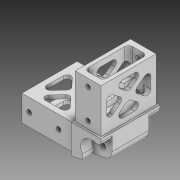
# Autodesk Inventor part: 254 Billet Bottom Block
Saved by Autodesk Inventor 2021 (Build 250183000, 183)
## iProperties
Created: 2021-03-21
Part Number: 254 Billet Bottom Block
Material: Generic
Document SubType Name: Modeling
Density: 1 g/cm^3
Appearance: Default
Autodesk Inventor part; units mm, degrees
ref_plane "YZ Plane" through (0, 0, 0) normal (1, 0, 0) x (0, 1, 0)
ref_plane "XZ Plane" through (0, 0, 0) normal (0, 1, 0) x (-1, 0, 0)
ref_plane "XY Plane" through (0, 0, 0) normal (0, 0, 1) x (1, 0, 0)
sketch "Sketch1" plane through (0, 0, 0) normal (0, 0, 1) x (1, 0, 0)
  line L0 (-71.4375, 14.2875) -> (-26.9875, 14.2875)
  line L1 (-26.9875, 14.2875) -> (-26.9875, -11.1125)
  line L2 (-26.9875, -11.1125) -> (-71.4375, -11.1125)
  line L3 (-71.4375, -11.1125) -> (-71.4375, 14.2875)
  line L4 (-26.9875, 14.2875) -> (-1.5875, 14.2875)
  line L5 (-1.5875, 14.2875) -> (-1.5875, 52.3875)
  line L6 (-1.5875, 52.3875) -> (-26.9875, 52.3875)
  line L7 (-26.9875, 52.3875) -> (-26.9875, 14.2875)
  circle A0 centre (-39.6875, 1.5875) radius 2.0193
  circle A1 centre (-65.0875, 1.5875) radius 2.0193
  circle A2 centre (-14.2875, 20.6375) radius 2.0193
  circle A3 centre (-14.2875, 46.0375) radius 2.0193
  line L8 (0, 0) -> (0, 64.1465) construction
  circle A4 centre (-9.525, 0) radius 9.525 construction
  line L9 (-31.5382, -9.525) -> (14.8852, -9.525) construction
  circle A5 centre (-9.525, 0) radius 2.5527
  arc A6 (-8.1574, -7.8188) -> (-1.5875, 0) centre (-9.525, 0) ccw
  line L10 (-1.5875, 14.2875) -> (-1.5875, 0)
  line L11 (-26.9875, -11.1125) -> (-8.1574, -7.8188)
  line L12 (-25.4, 52.3875) -> (-25.4, 17.5252)
  line L13 (-25.4, 17.5252) -> (-25.4, 14.2875)
  line L14 (-71.4375, 12.7) -> (-26.9875, 12.7)
  line L15 (-3.175, 14.2875) -> (-3.175, 52.3875)
  line L16 (-26.9875, -9.525) -> (-71.4375, -9.525)
  point P0 (-71.4375, 1.5875)
  point P1 (-14.2875, 14.2875)
  dimension "d0" = 4.0386
  dimension "d3" = 25.4
  dimension "d8" = 6.35
  dimension "d9" = 12.7
  dimension "d10" = 25.4
  dimension "d13" = 25.4
  dimension "d18" = 6.35
  dimension "d19" = 6.35
  dimension "d20" = 19.05
  dimension "d21" = 1.5875
  dimension "d22" = 1.5875
  dimension "d23" = 5.1054
  dimension "d24" = 15.875
  dimension "d25" = 1.5875
  dimension "d26" = 1.5875
  dimension "d27" = 1.5875
  dimension "d28" = 1.5875
  constraints: 34 end point, 9 point on line, 7 centre point, 6 perpendicular, 4 horizontal, 4 parallel, 4 tangent, 3 vertical, 2 horizontal alignment, 2 midpoint, 2 point on circle, 1 coincident, 1 equal radius, 1 vertical alignment, 4 other
  measures "d0" diameter of A0
  measures "d3" distance of A0.centre A1.centre
  measures "d8" distance from line of A1.centre L3
  measures "d9" distance from line of L1 A0.centre
  measures "d10" distance of L2.end L0.start
  measures "d13" distance of A2.centre A3.centre
  measures "d18" distance from line of L4 A2.centre
  measures "d19" distance from line of L6 A3.centre
  measures "d20" diameter of A4
  measures "d21" distance between parallel lines of L2 L9
  measures "d22" distance between parallel lines of L8 L5
  measures "d23" diameter of A5
  measures "d24" diameter of A6
  measures "d25" distance between parallel lines of L7 L12
  measures "d26" distance between parallel lines of L0 L14
  measures "d27" distance between parallel lines of L2 L16
  measures "d28" distance between parallel lines of L5 L15
extrude "Extrusion1" add sketch "Sketch1" along normal mid plane 50.8 contours L4 L10 A6 L11 L1 | L14 L1 L16 L3 | L13 L12 L6 L15 L4
sketch "Sketch2" plane through (0, 0, 25.4) normal (0, 0, 1) x (1, 0, 0)
  circle A0 centre (-9.525, 0) radius 2.5527 projected
  circle A1 centre (-9.525, 0) radius 9.6044
  point P0 (0, 0)
  dimension "d31" = 19.2087
  constraints: 1 centre point, 1 coincident
  measures "d31" diameter of A1
extrude "Extrusion2" cut sketch "Sketch2" against normal blind 9.525
mirror "Mirror1" about plane through (0, 0, 0) normal (0, 0, 1) of "Extrusion2"
fillet "Fillet1" radius 3.175 4 edges at (-13.4839, -8.7505, 20.6375) (-1.5875, 5.4074, 20.6375) (-1.5875, 5.4074, -20.6375) (-13.4839, -8.7505, -20.6375)
sketch "Sketch3" plane through (-71.4375, -9.525, 25.4) normal (-1, 0, 0) x (0, 0, 1)
  line L0 (-50.8, 0) -> (0, 0) projected
  line L1 (0, 22.225) -> (0, 0) projected
  line L2 (-50.8, 22.225) -> (0, 22.225) projected
  line L3 (-50.8, 0) -> (-50.8, 22.225) projected
  line L4 (-44.45, 19.05) -> (-6.35, 19.05)
  line L5 (-6.35, 19.05) -> (-6.35, 3.175)
  line L6 (-6.35, 3.175) -> (-44.45, 3.175)
  line L7 (-44.45, 3.175) -> (-44.45, 19.05)
  line L8 (-49.2125, 22.225) -> (-49.2125, 0)
  line L9 (0, 0) -> (-50.8, 0) projected
  line L10 (-50.8, 22.225) -> (0, 22.225) projected
  line L11 (-1.5875, 22.225) -> (-1.5875, 0)
  point P0 (-25.4, 9.525)
  point P1 (-49.2125, 0)
  dimension "d35" = 6.35
  dimension "d36" = 6.35
  dimension "d37" = 3.175
  dimension "d38" = 3.175
  dimension "d49" = 1.5875
  dimension "d50" = 1.5875
  constraints: 12 end point, 4 point on line, 3 parallel, 1 horizontal, 1 perpendicular, 1 vertical
  measures "d35" distance between parallel lines of L1 L5
  measures "d36" distance between parallel lines of L3 L7
  measures "d37" distance between parallel lines of L2 L4
  measures "d38" distance between parallel lines of L0 L6
  measures "d49" distance between parallel lines of L3 L8
  measures "d50" distance between parallel lines of L1 L11
extrude "Extrusion3" cut sketch "Sketch3" against normal up to surface (44.45 mm away) contours L3 L2 L8 L0 | L11 L2 L1 L0 | L4 L5 L6 L7
sketch "Sketch4" plane through (-25.4, 52.3875, 25.4) normal (0, 1, 0) x (1, 0, 0)
  line L0 (0, 50.8) -> (0, 0) projected
  line L1 (22.225, 0) -> (0, 0) projected
  line L2 (22.225, 50.8) -> (22.225, 0) projected
  line L3 (0, 50.8) -> (22.225, 50.8) projected
  line L4 (19.05, 6.35) -> (3.175, 6.35)
  line L5 (3.175, 6.35) -> (3.175, 44.45)
  line L6 (3.175, 44.45) -> (19.05, 44.45)
  line L7 (19.05, 44.45) -> (19.05, 6.35)
  line L8 (22.225, 49.2125) -> (0, 49.2125)
  line L9 (22.225, 1.5875) -> (0, 1.5875)
  point P0 (25.4, 25.4)
  dimension "d41" = 3.175
  dimension "d42" = 3.175
  dimension "d43" = 6.35
  dimension "d44" = 6.35
  dimension "d45" = 1.5875
  dimension "d46" = 1.5875
  constraints: 12 end point, 4 point on line, 3 perpendicular, 2 parallel, 1 horizontal
  measures "d41" distance between parallel lines of L2 L7
  measures "d42" distance between parallel lines of L0 L5
  measures "d43" distance between parallel lines of L1 L4
  measures "d44" distance between parallel lines of L3 L6
  measures "d45" distance between parallel lines of L1 L9
  measures "d46" distance between parallel lines of L3 L8
extrude "Extrusion4" cut sketch "Sketch4" against normal up to surface (38.1 mm away) contours L3 L2 L8 L0 | L9 L2 L1 L0 | L4 L5 L6 L7
sketch "Sketch5" plane through (-71.4375, 12.7, 23.8125) normal (0, 1, 0) x (1, 0, 0)
  line L0 (0, 0) -> (44.45, 0) projected
  line L1 (44.45, 47.625) -> (44.45, 0) projected
  line L2 (44.45, 47.625) -> (0, 47.625) projected
  line L3 (0, 47.625) -> (0, 0) projected
  line L4 (44.45, 4.7625) -> (44.45, 42.8625) projected
  line L5 (0, 42.8625) -> (44.45, 42.8625) projected
  line L6 (0, 4.7625) -> (0, 42.8625) projected
  line L7 (0, 4.7625) -> (44.45, 4.7625) projected
  line L8 (4.7625, 0) -> (4.7625, 47.625)
  line L9 (39.6875, 0) -> (39.6875, 47.625)
  line L10 (44.45, 47.625) -> (0, 47.625) projected
  line L11 (0, 4.7625) -> (44.45, 4.7625) projected
  line L12 (39.6875, 4.7625) -> (4.7625, 42.8625) construction
  line L13 (41.4428, 6.3716) -> (6.5178, 44.4716)
  line L14 (3.0072, 41.2534) -> (37.9322, 3.1534)
  arc A0 (37.9322, 3.1534) -> (41.4428, 6.3716) centre (39.6875, 4.7625) ccw
  arc A1 (6.5178, 44.4716) -> (3.0072, 41.2534) centre (4.7625, 42.8625) ccw
  line L15 (4.7625, 4.7625) -> (39.6875, 42.8625) construction
  line L16 (6.5178, 3.1534) -> (41.4428, 41.2534)
  line L17 (37.9322, 44.4716) -> (3.0072, 6.3716)
  arc A2 (3.0072, 6.3716) -> (6.5178, 3.1534) centre (4.7625, 4.7625) ccw
  arc A3 (41.4428, 41.2534) -> (37.9322, 44.4716) centre (39.6875, 42.8625) ccw
  point P0 (71.4375, 23.8125)
  point P1 (22.225, 23.8125)
  point P2 (22.225, 23.8125)
  point P3 (22.225, 27.3365)
  point P4 (36.4572, 42.8625)
  point P5 (7.9928, 42.8625)
  point P6 (39.6875, 39.3385)
  point P7 (25.4553, 23.8125)
  point P8 (39.6875, 8.2865)
  point P9 (22.225, 20.2885)
  point P10 (7.9928, 4.7625)
  point P11 (36.4572, 4.7625)
  point P12 (4.7625, 8.2865)
  point P13 (18.9947, 23.8125)
  point P14 (4.7625, 39.3385)
  dimension "d52" = 4.7625
  dimension "d53" = 4.7625
  dimension "d54" = 4.7625
  dimension "d55" = 4.7625
  constraints: 20 end point, 12 point on line, 8 point on circle, 8 tangent, 4 centre point, 2 midpoint, 2 parallel, 2 perpendicular
  measures "d52" distance between parallel lines of L3 L8
  measures "d53" distance between parallel lines of L1 L9
  measures "d54" diameter of A1
  measures "d55" diameter of A3
extrude "Extrusion5" cut sketch "Sketch5" against normal through all contours L16 L14 L7 | L8 L14 L17 | L13 L16 L9 | L5 L17 L13
sketch "Sketch7" plane through (-25.4, 14.2875, -23.8125) normal (-1, 0, 0) x (0, 0, 1)
  line L0 (0, 38.1) -> (0, 0) projected
  line L1 (0, 0) -> (47.625, 0) projected
  line L2 (47.625, 0) -> (47.625, 38.1) projected
  line L3 (0, 38.1) -> (47.625, 38.1) projected
  line L4 (4.7625, 0) -> (42.8625, 0) projected
  line L5 (42.8625, 38.1) -> (42.8625, 0) projected
  line L6 (4.7625, 38.1) -> (42.8625, 38.1) projected
  line L7 (4.7625, 38.1) -> (4.7625, 0) projected
  line L8 (47.625, 33.3375) -> (0, 33.3375)
  line L9 (47.625, 4.7625) -> (0, 4.7625)
  line L10 (0, 8.3693) -> (0, 4.3307) projected
  line L11 (42.8625, 33.7693) -> (42.8625, 29.7307) projected
  line L12 (42.8625, 33.3375) -> (4.7625, 4.7625) construction
  line L13 (4.7625, 4.3307) -> (4.7625, 8.3693) projected
  line L14 (41.4337, 35.2425) -> (3.3338, 6.6675)
  line L15 (6.1913, 2.8575) -> (44.2912, 31.4325)
  arc A0 (44.2912, 31.4325) -> (41.4337, 35.2425) centre (42.8625, 33.3375) ccw
  arc A1 (3.3338, 6.6675) -> (6.1913, 2.8575) centre (4.7625, 4.7625) ccw
  line L16 (4.7625, 29.7307) -> (4.7625, 33.7693) projected
  line L17 (4.7625, 33.3375) -> (42.8625, 4.7625) construction
  line L18 (3.3338, 31.4325) -> (41.4337, 2.8575)
  line L19 (44.2912, 6.6675) -> (6.1913, 35.2425)
  arc A2 (6.1913, 35.2425) -> (3.3338, 31.4325) centre (4.7625, 33.3375) ccw
  arc A3 (41.4337, 2.8575) -> (44.2912, 6.6675) centre (42.8625, 4.7625) ccw
  point P0 (23.8125, -14.2875)
  point P1 (23.8125, 19.05)
  point P2 (23.8125, 19.05)
  point P3 (8.7312, 33.3375)
  point P4 (23.8125, 22.0266)
  point P5 (38.8937, 33.3375)
  point P6 (19.8438, 19.05)
  point P7 (4.7625, 30.3609)
  point P8 (4.7625, 7.7391)
  point P9 (38.8937, 4.7625)
  point P10 (23.8125, 16.0734)
  point P11 (8.7313, 4.7625)
  point P12 (27.7812, 19.05)
  point P13 (42.8625, 7.7391)
  point P14 (42.8625, 30.3609)
  dimension "d59" = 4.7625
  dimension "d60" = 4.7625
  dimension "d61" = 4.7625
  dimension "d62" = 4.7625
  constraints: 20 end point, 12 point on line, 8 point on circle, 8 tangent, 4 centre point, 3 parallel, 2 midpoint, 1 perpendicular
  measures "d59" distance between parallel lines of L3 L8
  measures "d60" distance between parallel lines of L1 L9
  measures "d61" diameter of A1
  measures "d62" diameter of A3
extrude "Extrusion6" cut sketch "Sketch7" against normal through all contours L18 L14 L7 | L8 L14 L19 | L15 L18 L9 | L15 L5 L19
fillet "Fillet3" radius 3.302 47 edges at (-31.75, 11.1125, -15.526) (-45.9822, 11.1125, 0) (-45.9822, -7.9375, 0) (-31.75, -7.9375, -15.526) (-31.75, 11.1125, 15.526) (-31.75, -7.9375, 15.526) (-49.2125, 11.1125, 3.524) (-49.2125, -7.9375, 3.524) (-49.2125, 11.1125, -3.524) (-49.2125, -7.9375, -3.524) (-66.675, 11.1125, 15.526) (-52.4428, 11.1125, 0) (-52.4428, -7.9375, 0) (-66.675, -7.9375, 15.526) (-66.675, 11.1125, -15.526) (-66.675, -7.9375, -15.526) (-34.9803, 11.1125, 19.05) (-63.4447, 11.1125, 19.05) (-34.9803, -7.9375, 19.05) (-63.4447, -7.9375, 19.05) (-34.9803, 11.1125, -19.05) (-63.4447, 11.1125, -19.05) (-34.9803, -7.9375, -19.05) (-23.8125, 33.3375, -3.9687) (-4.7625, 33.3375, -3.9687) (-4.7625, 30.3609, 0) (-4.7625, 19.05, 15.0812) (-4.7625, 19.05, -15.0812) (-23.8125, 30.3609, 0) (-23.8125, 19.05, -15.0812) (-23.8125, 19.05, 15.0812) (-4.7625, 36.3141, 0) (-4.7625, 47.625, -15.0812) (-4.7625, 47.625, 15.0812) (-23.8125, 36.3141, 0) (-23.8125, 47.625, 15.0812) (-23.8125, 47.625, -15.0812) (-23.8125, 33.3375, 3.9687) (-4.7625, 33.3375, 3.9687) (-23.8125, 44.6484, 19.05) (-23.8125, 44.6484, -19.05) (-23.8125, 22.0266, -19.05) (-4.7625, 44.6484, 19.05) (-4.7625, 22.0266, 19.05) (-23.8125, 22.0266, 19.05) (-4.7625, 44.6484, -19.05) (-4.7625, 22.0266, -19.05)
fillet "Fillet2" radius 3.302 31 edges at (-59.6916, 9.525, -19.05) (-67.4411, 9.525, -19.05) (-38.7334, 9.525, -19.05) (-30.9839, 9.525, -19.05) (-67.4411, -6.35, -19.05) (-30.9839, -6.35, -19.05) (-38.7334, -6.35, -19.05) (-59.6916, 9.525, 19.05) (-67.4411, 9.525, 19.05) (-38.7334, 9.525, 19.05) (-30.9839, 9.525, 19.05) (-67.4411, -6.35, 19.05) (-59.6916, -6.35, 19.05) (-30.9839, -6.35, 19.05) (-38.7334, -6.35, 19.05) (-22.225, 41.3464, -19.05) (-22.225, 48.518, -19.05) (-22.225, 25.3286, -19.05) (-22.225, 18.157, -19.05) (-6.35, 48.518, -19.05) (-6.35, 41.3464, -19.05) (-6.35, 18.157, -19.05) (-6.35, 25.3286, -19.05) (-6.35, 48.518, 19.05) (-6.35, 41.3464, 19.05) (-6.35, 18.157, 19.05) (-6.35, 25.3286, 19.05) (-22.225, 41.3464, 19.05) (-22.225, 48.518, 19.05) (-22.225, 25.3286, 19.05) (-22.225, 18.157, 19.05)
equation "\"d18\" = d8"
equation "\"d19\" = d18"
equation "\"d26\" = d25"
equation "\"d27\" = d26"
equation "\"d28\" = d25"
equation "\"d36\" = d35"
equation "\"d38\" = d37"
equation "\"d50\" = d49"
equation "\"d44\" = d43"
equation "\"d46\" = d45"
equation "\"d53\" = d52"
equation "\"d60\" = d59"
body "Solid1"
